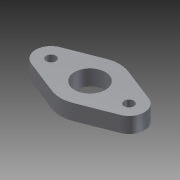
# Autodesk Inventor part: fixador barra
Saved by Autodesk Inventor 2012 (Build 160160000, 160)
## iProperties
Created: 2014-12-16
Part Number: fixador barra
Material: Default
Document SubType Name: Modeling
Designer: PRINCIPAL
Density: 1 g/cm^3
Author: PRINCIPAL
Autodesk Inventor part; units mm, degrees
ref_plane "YZ Plane" through (0, 0, 0) normal (1, 0, 0) x (0, 1, 0)
ref_plane "XZ Plane" through (0, 0, 0) normal (0, 1, 0) x (-1, 0, 0)
ref_plane "XY Plane" through (0, 0, 0) normal (0, 0, 1) x (1, 0, 0)
sketch "Boceto1" plane through (0, 0, 0) normal (0, 0, 1) x (1, 0, 0)
  arc A0 (12.5, 1.55) -> (10.95, 0) centre (12.5, 0) ccw
  arc A1 (10.95, 0) -> (12.5, -1.55) centre (12.5, 0) ccw
  arc A2 (12.5, -1.55) -> (14.05, 0) centre (12.5, 0) ccw
  arc A3 (14.05, 0) -> (12.5, 1.55) centre (12.5, 0) ccw
  arc A4 (0, 4.95) -> (-4.95, 0) centre (0, 0) ccw
  arc A5 (-4.95, 0) -> (0, -4.95) centre (0, 0) ccw
  arc A6 (0, -4.95) -> (4.95, 0) centre (0, 0) ccw
  arc A7 (4.95, 0) -> (0, 4.95) centre (0, 0) ccw
  arc A8 (-12.5, 1.55) -> (-14.05, 0) centre (-12.5, 0) ccw
  arc A9 (-14.05, 0) -> (-12.5, -1.55) centre (-12.5, 0) ccw
  arc A10 (-12.5, -1.55) -> (-10.95, 0) centre (-12.5, 0) ccw
  arc A11 (-10.95, 0) -> (-12.5, 1.55) centre (-12.5, 0) ccw
  arc A12 (3.4398, 8.8017) -> (-3.4398, 8.8017) centre (0, 0) ccw
  line L0 (-3.4398, 8.8017) -> (-14.2836, 4.5639)
  arc A13 (-14.2836, 4.5639) -> (-14.2836, -4.5639) centre (-12.5, 0) ccw
  line L1 (-14.2836, -4.5639) -> (-3.4398, -8.8017)
  arc A14 (-3.4398, -8.8017) -> (3.4398, -8.8017) centre (0, 0) ccw
  line L2 (3.4398, -8.8017) -> (14.2836, -4.5639)
  arc A15 (14.2836, -4.5639) -> (14.2836, 4.5639) centre (12.5, 0) ccw
  line L3 (14.2836, 4.5639) -> (3.4398, 8.8017)
  point P0 (0, 0)
  constraints: 32 point on circle, 16 centre point, 8 end point
extrude "Extrusión1" add sketch "Boceto1" along normal blind 5
